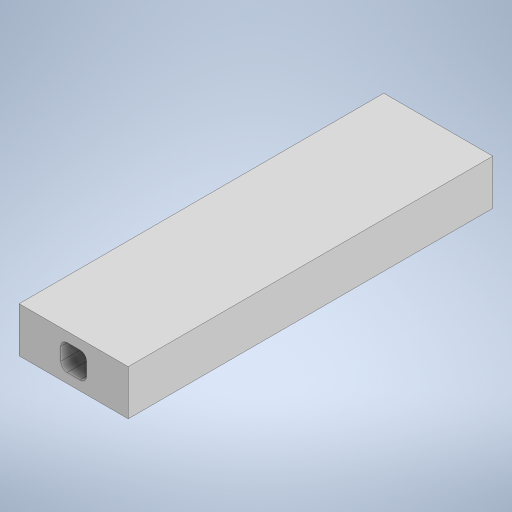
# Autodesk Inventor part: 막대마지막
Saved by Autodesk Inventor 2023 (Build 270158000, 158)
## iProperties
Created: 2023-05-17
Part Number: 막대마지막
Material: 일반
Document SubType Name: Modeling
Designer: rlatk
Density: 1 g/cm^3
Appearance: 기본값
Author: rlatk
Autodesk Inventor part; units mm, degrees
ref_plane "YZ Plane" through (0, 0, 0) normal (1, 0, 0) x (0, 1, 0)
ref_plane "XZ Plane" through (0, 0, 0) normal (0, 1, 0) x (-1, 0, 0)
ref_plane "XY Plane" through (0, 0, 0) normal (0, 0, 1) x (1, 0, 0)
sketch "스케치1" plane through (0, 0, 0) normal (0, 1, 0) x (-1, 0, 0)
  line L0 (0, 0) -> (-16.9, 0)
  line L1 (-16.9, 0) -> (-16.9, -56.5)
  line L2 (-16.9, -56.5) -> (0, -56.5)
  line L3 (0, -56.5) -> (0, 0)
  dimension "d0" = 16.9
  dimension "d1" = 56.5
  constraints: 8 end point, 2 parallel, 1 horizontal, 1 perpendicular
  measures "d0" distance of L2.end L1.end
  measures "d1" distance of L1.end L0.end
extrude "돌출1" add sketch "스케치1" along normal blind 7
sketch "스케치2" plane through (0, 0, 0) normal (0, 0, 1) x (1, 0, 0)
  line L0 (16.9, 7) -> (0, 7) projected
  line L1 (8.45, 5.5) -> (8.45, 1.5)
  line L2 (16.9, 0) -> (0, 0) projected
  line L3 (6.45, 5.5) -> (6.45, 1.5)
  line L4 (10.45, 5.5) -> (10.45, 1.5)
  line L5 (6.45, 5.5) -> (10.45, 5.5)
  line L6 (6.45, 1.5) -> (10.45, 1.5)
  dimension "d4" = 2
  dimension "d5" = 2
  dimension "d6" = 1.5
  dimension "d7" = 1.5
  constraints: 10 end point, 3 perpendicular, 2 midpoint, 1 vertical
  measures "d4" distance between parallel lines of L3 L1
  measures "d5" distance between parallel lines of L1 L4
  measures "d6" distance between parallel lines of L6 L2
  measures "d7" distance between parallel lines of L5 L0
extrude "돌출3" cut sketch "스케치2" against normal blind 56.5
fillet "모깎기1" radius 1 4 edges at (6.45, 5.5, -28.25) (6.45, 1.5, -28.25) (10.45, 1.5, -28.25) (10.45, 5.5, -28.25)
